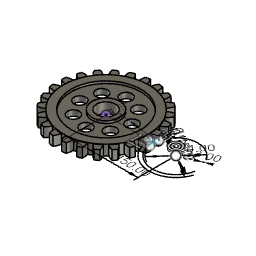
Planetary gear v1 (Autodesk Fusion 360 design; units mm, degrees)
Autodesk Fusion 360 part; units mm, degrees
sketch "Sketch1" plane through (0, 0, 0) normal (0, 0, 1) x (1, 0, 0)
  line L0 (87.8446, -25.6044) -> (90.2447, -26.3039)
  arc A0 (91.1595, -7.8859) -> (91.1595, 7.8859) centre (0, 0) ccw
  arc A1 (104.8992, -4.5995) -> (104.8992, 4.5995) centre (0, 0) ccw
  arc A2 (104.8992, 4.5995) -> (91.1595, 7.8859) centre (90.2447, -26.3039) ccw
  arc A3 (91.1595, -7.8859) -> (104.8992, -4.5995) centre (90.2447, 26.3039) ccw
  circle A4 centre (0, 0) radius 91.5
  dimension "d1" = 183
  dimension "d4" = 210
  dimension "d9" = 183
  constraint coincident A0.centre A1.centre
  measures "d1" diameter of A0
  measures "d4" diameter of A1
  measures "d9" diameter of A4
extrude "Extrude1" add sketch "Sketch1" along normal mid plane 20 contours A0 A1 A2 A3 A4 makes body 1
extrude "Extrude2" add sketch "Sketch1" along normal mid plane 22 contours A0 A4 bodies 1
sketch "Sketch2" plane through (0, 0, 11) normal (0, 0, 1) x (-1, 0, 0)
  circle A0 centre (0, 0) radius 91.5
  circle A1 centre (0, 0) radius 20
  circle A2 centre (0, 0) radius 30
  circle A3 centre (0, 0) radius 75
  circle A4 centre (0, -50) radius 12.5
  dimension "d14" = 40
  dimension "d15" = 60
  dimension "d16" = 150
  dimension "d17" = 25
  dimension "d18" = 50
  constraint coincident A0.centre A1.centre
  constraint concentric A1 A2
  constraint concentric A1 A3
  measures "d14" diameter of A1
  measures "d15" diameter of A2
  measures "d16" diameter of A3
  measures "d17" diameter of A4
  measures "d18" distance of A0.centre A4.centre
extrude "Extrude3" cut sketch "Sketch2" against normal blind 100 contours A1 bodies 1
extrude "Extrude4" cut sketch "Sketch2" against normal blind 40 contours A4 bodies 1
extrude "Extrude5" cut sketch "Sketch2" against normal blind 5 contours A3 bodies 1
pattern_circular "C-Pattern1" count 8 over 360 about axis through (0, 0, 11) along (0, 0, 1) of "Extrude4"
mirror "Mirror1" about plane through (0, 0, 0) normal (0, 0, 1) of "Extrude5"
pattern_circular "C-Pattern2" count 24 over 360 about axis through (0, 0, 11) along (0, 0, 1) of "Extrude1" makes body 2 at (87.1458, 27.8901, -3.3333) makes body 3 at (81.3427, 41.9001, 3.3333) makes body 4 at (60.2155, 68.8937, 3.3333) makes body 5 at (41.9001, 81.3427, 3.3333) makes body 6 at (27.8901, 87.1458, 3.3333) makes body 7 at (0.8773, 91.4958, -3.3333) makes body 8 at (-24.5282, 88.1511, 3.3333) makes body 9 at (-40.3327, 82.1311, -3.3333) makes body 10 at (-68.8937, 60.2155, 3.3333) makes body 11 at (-82.1311, 40.3327, -3.3333) makes body 12 at (-86.595, 29.556, -3.3333) makes body 13 at (-91.4958, 0.8773, -3.3333) makes body 14 at (-88.1511, -24.5282, 3.3333) makes body 15 at (-82.1311, -40.3327, -3.3333) makes body 16 at (-60.2155, -68.8937, 3.3333) makes body 17 at (-44.9881, -79.6763, 3.3333) makes body 18 at (-27.8901, -87.1458, 3.3333) makes body 19 at (-0.8773, -91.4958, -3.3333) makes body 20 at (22.8335, -88.6052, -3.3333) makes body 21 at (41.9001, -81.3427, 3.3333) makes body 22 at (68.8937, -60.2155, 3.3333) makes body 23 at (79.6763, -44.9881, 3.3333) makes body 24 at (88.6052, -22.8335, 3.3333)
combine "Combine1" operation add target body 1 tool bodies 14 4 8 23 2 6 17 19 9 5 20 3 18 16 22 21 11 12 10 24 13 15 7
sketch "Sketch3" plane through (0, 0, 0) normal (0, 0, 1) x (1, 0, 0)
  circle A0 centre (150, 0) radius 50
  dimension "d31" = 100
  dimension "d32" = 150
  measures "d31" diameter of A0
  measures "d32" distance of origin A0.centre
move_body "Move1" bodies 1 to x (0.991445, 0.130526, 0) y (-0.130526, 0.991445, 0) z (0, 0, 1) at (0, 0, 0)
sketch "Sketch4" plane through (0, 0, 0) normal (0, 0, 1) x (1, 0, 0)
  line L0 (90.3678, 0) -> (106, 0)
  line L1 (106.3764, 5.7432) -> (100.4278, 6.5263)
  arc A0 (92.5512, 2.4267) -> (92.5512, -2.4267) centre (150, 0) ccw
  arc A1 (106.3764, 5.7432) -> (106.5221, -6.758) centre (150, 0) ccw
  arc A2 (103.4021, 6.1347) -> (103.5119, -6.9177) centre (150, 0) ccw
  arc A3 (100.4278, 6.5263) -> (100.4278, -6.5263) centre (150, 0) ccw
  arc A4 (92.5512, 2.4267) -> (92.5512, -2.4267) centre (150, 0) ccw
  arc A5 (106.5221, 6.758) -> (106.5221, -6.758) centre (150, 0) ccw
  arc A6 (92.5512, -2.4267) -> (106.5221, -6.758) centre (104.1141, 10.1727) ccw
  arc A7 (103.5119, 6.9177) -> (103.5119, -6.9177) centre (150, 0) ccw
  arc A8 (100.4278, 6.5263) -> (100.4278, -6.5263) centre (150, 0) ccw
  arc A9 (106.5221, 6.758) -> (92.5512, 2.4267) centre (104.1141, -10.1727) ccw
  dimension "d34" = 150
  dimension "d39" = 7.5
  dimension "d40" = 100
  dimension "d41" = 115
  dimension "d42" = 94
  dimension "d43" = 3
  constraint concentric A1 A3
  constraint concentric A1 A2
  constraint concentric A0 A3
  constraint horizontal L0
  constraint coincident L1 A2.start
  constraint concentric A3 A8
  constraint concentric A3 A4
  constraint concentric A4 A7
  constraint concentric A2 A5
  constraint coincident L1.end A9
  constraint symmetric L0 A6 A9
  constraint coincident A1 L0.end
  constraint coincident A7.start A9
  constraint coincident A6 A3.end
  constraint coincident A6 A2.end
  measures "d34" distance of origin A0.centre
  measures "d39" angle of L0 L1
  measures "d40" diameter of A8
  measures "d41" diameter of A4
  measures "d42" diameter of A7
  measures "d43" distance of A5 A7
equation "d39 = ( 7.5 ) * 1 deg"
